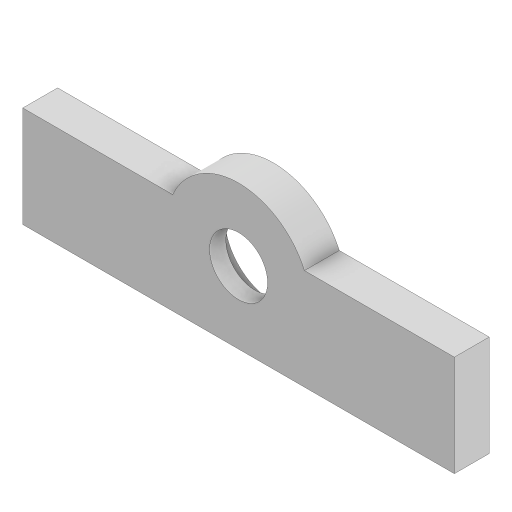
# Autodesk Inventor part: AOPORTE DE CAJA SEPARADORA
Saved by Autodesk Inventor 2024 (Build 280153000, 153)
## iProperties
Created: 2024-06-16
Part Number: AOPORTE DE CAJA SEPARADORA
Material: Generic
Document SubType Name: Modeling
Designer: Jhuliams
Density: 1 g/cm^3
Appearance: Default
Author: Jhuliams
Autodesk Inventor part; units mm, degrees
ref_plane "YZ Plane" through (0, 0, 0) normal (1, 0, 0) x (0, 1, 0)
ref_plane "XZ Plane" through (0, 0, 0) normal (0, 1, 0) x (-1, 0, 0)
ref_plane "XY Plane" through (0, 0, 0) normal (0, 0, 1) x (1, 0, 0)
sketch "Sketch1" plane through (0, 0, 0) normal (0, 0, 1) x (1, 0, 0)
  line L0 (93, 12.5) -> (93, -12.5)
  line L1 (93, -12.5) -> (28.3681, -12.5)
  line L2 (-93, -12.5) -> (-93, 12.5)
  line L3 (-93, 12.5) -> (30.7237, -4.1295) construction
  line L4 (93, 12.5) -> (-93, -12.5) construction
  line L5 (28.3681, -12.5) -> (93, -12.5)
  line L6 (93, -12.5) -> (93, -31)
  line L7 (93, -31) -> (-93, -31)
  line L8 (-93, -31) -> (-93, -12.5)
  arc A0 (28.3681, 12.5) -> (-28.3681, 12.5) centre (0, 0) ccw
  circle A1 centre (0, 0) radius 12.5
  line L9 (-93, 12.5) -> (-28.3681, 12.5)
  line L10 (28.3681, 12.5) -> (93, 12.5)
  dimension "d1" = 186
  dimension "d2" = 25
  dimension "d5" = 25
  constraints: 22 end point, 5 parallel, 3 horizontal, 3 perpendicular, 2 centre point, 2 coincident, 2 point on circle, 1 midpoint, 1 point on line
  measures "d1" distance of L0.end L2.start
  measures "d2" distance of L0.start L0.end
  measures "d5" diameter of A1
extrude "Extrusion1" add sketch "Sketch1" along normal blind 15
sketch "Sketch2" plane through (0, 0, 0) normal (0, 0, -1) x (-1, 0, 0)
  circle A0 centre (0, 0) radius 21
  dimension "d6" = 42
  constraints: 1 centre point, 1 coincident
  measures "d6" diameter of A0
extrude "Extrusion2" cut sketch "Sketch2" against normal blind 8
body "Solid1"
